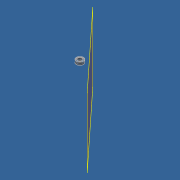
# Autodesk Inventor part: 6mm Wellen klemme
Saved by Autodesk Inventor 2014 SP2 (Build 180246200, 246)
## iProperties
Created: 2014-12-19
Part Number: 6mm Wellen klemme
Material: Stahl
Document SubType Name: Modeling
Designer: 4ndreas
Density: 7.85 g/cm^3
Appearance: Stahl
Mass: 1.50256 g
Surface Area: 3.07752 cm^2
Volume: 0.191408 cm^3
Author: 4ndreas
Autodesk Inventor part; units mm, degrees
ref_plane "YZ Plane" through (0, 0, 0) normal (1, 0, 0) x (0, 1, 0)
ref_plane "XZ Plane" through (0, 0, 0) normal (0, 1, 0) x (-1, 0, 0)
ref_plane "XY Plane" through (0, 0, 0) normal (0, 0, 1) x (1, 0, 0)
sketch "Skizze1" plane through (0, 0, 0) normal (0, 0, 1) x (1, 0, 0)
  circle A0 centre (0, 0) radius 3
  circle A1 centre (0, 0) radius 5
  dimension "d0" = 6
  dimension "d1" = 10
  constraints: 2 centre point, 2 coincident
  measures "d0" diameter of A0
  measures "d1" diameter of A1
extrude "Extrusion1" add sketch "Skizze1" against normal blind 4
ref_plane "Arbeitsebene1" through (42.4595, -31.8083, 21.313) normal (-0.7331838, -0.6800306, 0) x (-0.6800306, 0.7331838, 0)
sketch "Skizze2" plane through (42.4595, -31.8083, 21.313) normal (-0.7331838, -0.6800306, 0) x (-0.6800306, 0.7331838, 0)
  line L0 (57.1951, 25.313) -> (47.1951, 25.313) projected
  line L1 (57.1951, 21.313) -> (47.1951, 21.313) projected
  line L2 (57.1951, 21.313) -> (57.1951, 25.313) projected
  line L3 (47.1951, 21.313) -> (47.1951, 25.313) projected
  line L4 (52.1951, 117.2) -> (52.1951, -24.2)
  line L5 (57.1951, 25.313) -> (47.1951, 21.313) construction
  point P0 (52.1951, 21.313)
  point P1 (52.1951, 23.313)
  constraints: 4 end point, 1 midpoint, 1 point on line, 1 vertical, 2 other
hole "Bohrung1" at (6.9652, 6.4603, -2) direction (-0.7331838, -0.6800306, 0) diameter 2.459 end up to surface thread size "M3x0.5" class "6H" standard "ANSI Metric M Profile"
